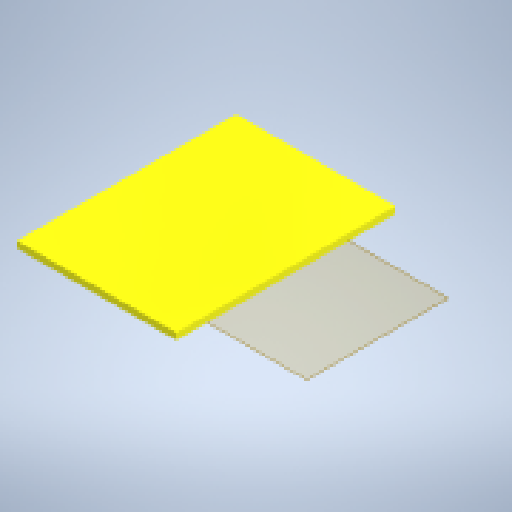
# Autodesk Inventor part: Sleed_Plate
Saved by Autodesk Inventor 2024 (Build 280153000, 153)
## iProperties
Created: 2023-11-25
Part Number: Sleed_Plate
Material: Generic
Document SubType Name: Modeling
Designer: danie
Density: 1 g/cm^3
Appearance: Default
Author: danie
Autodesk Inventor part; units mm, degrees
ref_plane "YZ Plane" through (0, 0, 0) normal (1, 0, 0) x (0, 1, 0)
ref_plane "XZ Plane" through (0, 0, 0) normal (0, 1, 0) x (-1, 0, 0)
ref_plane "XY Plane" through (0, 0, 0) normal (0, 0, 1) x (1, 0, 0)
ref_plane "Work Plane2" through (-92.9211, 111.7581, -85.645) normal (0, 1, 0) x (-1, 0, 0)
sketch "Sketch2" plane through (-92.9211, 111.7581, -85.645) normal (0, 1, 0) x (-1, 0, 0)
  line L0 (63, 0) -> (-63, 0)
  line L1 (-63, 0) -> (-63, -150)
  line L2 (-63, -150) -> (63, -150)
  line L3 (63, -150) -> (63, 0)
  line L4 (63, 0) -> (-63, -150) construction
  line L5 (-63, 0) -> (63, -150) construction
  line L6 (-114.9576, 160) -> (114.9576, 160)
  line L7 (114.9576, 160) -> (114.9576, -160)
  line L8 (114.9576, -160) -> (-114.9576, -160)
  line L9 (-114.9576, -160) -> (-114.9576, 160)
  line L10 (119.9576, -165) -> (119.9576, 165)
  line L11 (119.9576, 165) -> (-119.9576, 165)
  line L12 (-119.9576, 165) -> (-119.9576, 10)
  line L13 (-119.9576, -165) -> (119.9576, -165)
  line L14 (-119.9576, 10) -> (-114.9576, 10)
  line L15 (-114.9576, 10) -> (114.9576, 10)
  line L16 (114.9576, 10) -> (119.9576, 10)
  line L17 (-119.9576, 10) -> (-119.9576, -165)
  point P0 (-92.9211, 85.645)
  point P1 (0, -75)
  point P2 (114.9576, 160)
  dimension "d0" = 126
  dimension "d1" = 150
  dimension "d2" = 5
  dimension "d5" = 10
  dimension "d6" = 10
  constraints: 36 end point, 7 parallel, 6 perpendicular, 3 point on line, 2 horizontal, 2 midpoint, 4 other
  measures "d0" distance of L2.end L1.end
  measures "d1" distance of L1.end L0.end
  measures "d2" distance between parallel lines of L7 L10
  measures "d5" distance between parallel lines of L8 L2
  measures "d6" distance between parallel lines of L14 L0
extrude "Extrusion1" add sketch "Sketch2" along normal blind 10 contours L3 L2 L1 L0 | L15 L7 L8 L9 | L9 L8 L7 L16 L10 L13 L17 L14
body "Solid1"
